Autodesk Fusion 360 part; units mm, degrees
(part 5 of 5)
  spline S268 degree 5 poles (-42.5645, -20.3407) (-42.5479, -20.3413) (-42.5148, -20.3422) (-42.4652, -20.3436) (-42.3991, -20.3453) (-42.3165, -20.347) (-42.234, -20.3485) (-42.1516, -20.3496) (-42.0693, -20.3504) (-41.987, -20.3508) (-41.9048, -20.3509) (-41.8227, -20.3507) (-41.7407, -20.3502) (-41.6588, -20.3493) (-41.5769, -20.3481) (-41.4952, -20.3465) (-41.4135, -20.3446) (-41.332, -20.3423) (-41.2505, -20.3398) (-41.1691, -20.3368) (-41.0878, -20.3335) (-41.0211, -20.3305) (-40.9707, -20.3281) (-40.9365, -20.3264) (-40.9186, -20.3254) (-40.9168, -20.3254) knots -1 -1 -1 -1 -1 -1 -0.985714 -0.971429 -0.957143 -0.942857 -0.928571 -0.914286 -0.9 -0.885714 -0.871429 -0.857143 -0.842857 -0.828571 -0.814286 -0.8 -0.785714 -0.771429 -0.757143 -0.742857 -0.728571 -0.714286 -0.712736 -0.712736 -0.712736 -0.712736 -0.712736 -0.712736
  arc A171 (-31.978, -19.3309) -> (-30.8526, -21.1319) centre (0.7975, -0.1016) ccw
  spline S269 degree 5 poles (-45.622, -12.0047) (-45.6059, -12.0083) (-45.5735, -12.0154) (-45.525, -12.0261) (-45.4604, -12.0401) (-45.3796, -12.0573) (-45.2989, -12.0742) (-45.2181, -12.0907) (-45.1374, -12.1069) (-45.0566, -12.1228) (-44.9759, -12.1383) (-44.8953, -12.1534) (-44.8146, -12.1683) (-44.734, -12.1828) (-44.6533, -12.1969) (-44.5727, -12.2107) (-44.4922, -12.2241) (-44.4116, -12.2372) (-44.3311, -12.2499) (-44.2506, -12.2623) (-44.1702, -12.2743) (-44.1041, -12.2838) (-44.0541, -12.2909) (-44.0202, -12.2956) (-44.0024, -12.2981) (-44.0007, -12.2983) knots -1 -1 -1 -1 -1 -1 -0.985714 -0.971429 -0.957143 -0.942857 -0.928571 -0.914286 -0.9 -0.885714 -0.871429 -0.857143 -0.842857 -0.828571 -0.814286 -0.8 -0.785714 -0.771429 -0.757143 -0.742857 -0.728571 -0.714286 -0.712736 -0.712736 -0.712736 -0.712736 -0.712736 -0.712736
  spline S270 degree 3 poles (-42.826, -15.9134) (-42.7781, -15.8674) (-42.7397, -15.8125) (-42.6859, -15.6911) (-42.6712, -15.6257) (-42.6676, -15.4929) (-42.6788, -15.4268) (-42.7258, -15.3026) (-42.7613, -15.2457) (-42.852, -15.1487) (-42.9064, -15.1095) (-43.0219, -15.0565) (-43.0811, -15.0413) (-43.1416, -15.0368) knots 0 0 0 0 0.019923 0.019923 0.039846 0.039846 0.059769 0.059769 0.079691 0.079691 0.099614 0.099614 0.117812 0.117812 0.117812 0.117812
  arc A172 (-44.9524, -14.3096) -> (-44.7782, -14.8456) centre (0, 0) ccw
  circle A173 centre (-9.5671, -23.097) radius 1.5
  arc A174 (-45.7622, -11.4588) -> (-45.622, -12.0047) centre (0, 0) ccw
  spline S271 degree 5 poles (-43.7577, -17.628) (-43.7412, -17.6295) (-43.7082, -17.6326) (-43.6588, -17.6371) (-43.5929, -17.6429) (-43.5106, -17.6498) (-43.4284, -17.6564) (-43.3462, -17.6627) (-43.264, -17.6686) (-43.182, -17.6743) (-43.1, -17.6795) (-43.018, -17.6845) (-42.9361, -17.6891) (-42.8543, -17.6933) (-42.7726, -17.6973) (-42.6909, -17.7008) (-42.6093, -17.7041) (-42.5277, -17.707) (-42.4462, -17.7095) (-42.3648, -17.7117) (-42.2835, -17.7135) (-42.2168, -17.7147) (-42.1663, -17.7154) (-42.1321, -17.7158) (-42.1141, -17.716) (-42.1123, -17.7161) knots -1 -1 -1 -1 -1 -1 -0.985714 -0.971429 -0.957143 -0.942857 -0.928571 -0.914286 -0.9 -0.885714 -0.871429 -0.857143 -0.842857 -0.828571 -0.814286 -0.8 -0.785714 -0.771429 -0.757143 -0.742857 -0.728571 -0.714286 -0.712736 -0.712736 -0.712736 -0.712736 -0.712736 -0.712736
  spline S272 degree 5 poles (-45.6475, -1.9006) (-45.6491, -1.9013) (-45.6653, -1.9092) (-45.6961, -1.9241) (-45.7414, -1.9463) (-45.8013, -1.9758) (-45.8741, -2.0121) (-45.9468, -2.0487) (-46.0195, -2.0857) (-46.092, -2.123) (-46.1645, -2.1607) (-46.2369, -2.1987) (-46.3092, -2.2371) (-46.3814, -2.2758) (-46.4536, -2.3148) (-46.5256, -2.3542) (-46.5976, -2.3938) (-46.6694, -2.4339) (-46.7412, -2.4742) (-46.8129, -2.5149) (-46.8845, -2.5559) (-46.956, -2.5972) (-47.0132, -2.6305) (-47.056, -2.6556) (-47.0845, -2.6724) (-47.0988, -2.6809) knots 0.712736 0.712736 0.712736 0.712736 0.712736 0.712736 0.714286 0.728571 0.742857 0.757143 0.771429 0.785714 0.8 0.814286 0.828571 0.842857 0.857143 0.871429 0.885714 0.9 0.914286 0.928571 0.942857 0.957143 0.971429 0.985714 1 1 1 1 1 1
  line L83 (-26.7765, -11.9199) -> (-34.1296, -15.0714)
  arc A175 (36.5058, -13.0984) -> (37.1761, -11.0832) centre (0.7975, -0.1016) ccw
  arc A176 (27.48, -13.8145) -> (28.2723, -12.1489) centre (0.7975, -0.1016) ccw
  line L84 (29.5656, -8.6104) -> (37.1761, -11.0832)
  line L85 (28.2723, -12.1489) -> (35.5129, -15.556)
  line L86 (28.9883, -10.3622) -> (36.5058, -13.0984)
  arc A177 (30.6543, -3.0291) -> (30.7778, -1.1887) centre (0.7975, -0.1016) ccw
  line L87 (30.7778, -1.1887) -> (38.7642, -1.6912)
  spline S273 degree 5 poles (39.9814, -25.0393) (39.973, -25.025) (39.9561, -24.9965) (39.9307, -24.9539) (39.8967, -24.8972) (39.8539, -24.8265) (39.8109, -24.7561) (39.7677, -24.6859) (39.7242, -24.616) (39.6805, -24.5463) (39.6366, -24.4768) (39.5924, -24.4076) (39.548, -24.3387) (39.5033, -24.27) (39.4585, -24.2015) (39.4133, -24.1333) (39.368, -24.0654) (39.3224, -23.9978) (39.2765, -23.9304) (39.2305, -23.8632) (39.1841, -23.7964) (39.1459, -23.7416) (39.1168, -23.7004) (39.097, -23.6724) (39.0866, -23.6578) (39.0856, -23.6563) knots -1 -1 -1 -1 -1 -1 -0.985714 -0.971429 -0.957143 -0.942857 -0.928571 -0.914286 -0.9 -0.885714 -0.871429 -0.857143 -0.842857 -0.828571 -0.814286 -0.8 -0.785714 -0.771429 -0.757143 -0.742857 -0.728571 -0.714286 -0.712736 -0.712736 -0.712736 -0.712736 -0.712736 -0.712736
  spline S274 degree 5 poles (36.3835, -27.6324) (36.3852, -27.6328) (36.4027, -27.6371) (36.4359, -27.6452) (36.485, -27.657) (36.5499, -27.6725) (36.6292, -27.6909) (36.7085, -27.7091) (36.7881, -27.7269) (36.8678, -27.7444) (36.9476, -27.7615) (37.0277, -27.7784) (37.1078, -27.7949) (37.1881, -27.8111) (37.2686, -27.827) (37.3492, -27.8426) (37.4299, -27.8579) (37.5108, -27.8729) (37.5918, -27.8875) (37.673, -27.9019) (37.7543, -27.916) (37.8358, -27.9297) (37.901, -27.9405) (37.95, -27.9484) (37.9827, -27.9536) (37.9991, -27.9562) knots 0.712736 0.712736 0.712736 0.712736 0.712736 0.712736 0.714286 0.728571 0.742857 0.757143 0.771429 0.785714 0.8 0.814286 0.828571 0.842857 0.857143 0.871429 0.885714 0.9 0.914286 0.928571 0.942857 0.957143 0.971429 0.985714 1 1 1 1 1 1
  arc A178 (32.1518, -21.5703) -> (33.3022, -19.7852) centre (0.7975, -0.1016) ccw
  spline S275 degree 5 poles (38.3303, -27.5003) (38.3228, -27.4856) (38.3077, -27.4561) (38.285, -27.4119) (38.2546, -27.3532) (38.2164, -27.28) (38.1779, -27.207) (38.1392, -27.1342) (38.1002, -27.0617) (38.0609, -26.9894) (38.0214, -26.9173) (37.9817, -26.8455) (37.9417, -26.7739) (37.9015, -26.7025) (37.861, -26.6314) (37.8202, -26.5605) (37.7792, -26.4899) (37.738, -26.4195) (37.6964, -26.3493) (37.6547, -26.2794) (37.6126, -26.2098) (37.5779, -26.1528) (37.5514, -26.1098) (37.5335, -26.0807) (37.524, -26.0654) (37.5231, -26.0639) knots -1 -1 -1 -1 -1 -1 -0.985714 -0.971429 -0.957143 -0.942857 -0.928571 -0.914286 -0.9 -0.885714 -0.871429 -0.857143 -0.842857 -0.828571 -0.814286 -0.8 -0.785714 -0.771429 -0.757143 -0.742857 -0.728571 -0.714286 -0.712736 -0.712736 -0.712736 -0.712736 -0.712736 -0.712736
  spline S276 degree 5 poles (27.9562, -37.9991) (27.9536, -37.9827) (27.9484, -37.95) (27.9405, -37.901) (27.9297, -37.8358) (27.916, -37.7543) (27.9019, -37.673) (27.8875, -37.5918) (27.8729, -37.5108) (27.8579, -37.4299) (27.8426, -37.3492) (27.827, -37.2686) (27.8111, -37.1881) (27.7949, -37.1078) (27.7784, -37.0277) (27.7615, -36.9476) (27.7444, -36.8678) (27.7269, -36.7881) (27.7091, -36.7085) (27.6909, -36.6292) (27.6725, -36.5499) (27.657, -36.485) (27.6452, -36.4359) (27.6371, -36.4027) (27.6328, -36.3852) (27.6324, -36.3835) knots -1 -1 -1 -1 -1 -1 -0.985714 -0.971429 -0.957143 -0.942857 -0.928571 -0.914286 -0.9 -0.885714 -0.871429 -0.857143 -0.842857 -0.828571 -0.814286 -0.8 -0.785714 -0.771429 -0.757143 -0.742857 -0.728571 -0.714286 -0.712736 -0.712736 -0.712736 -0.712736 -0.712736 -0.712736
  spline S277 degree 3 poles (26.0639, -37.5231) (26.0074, -37.4881) (25.9447, -37.4645) (25.8136, -37.4427) (25.7466, -37.4446) (25.6171, -37.4742) (25.5559, -37.5014) (25.4473, -37.5779) (25.401, -37.6264) (25.3296, -37.7384) (25.3052, -37.8008) (25.2826, -37.9259) (25.2826, -37.987) (25.2933, -38.0467) knots 0 0 0 0 0.019923 0.019923 0.039846 0.039846 0.059769 0.059769 0.079691 0.079691 0.099614 0.099614 0.117812 0.117812 0.117812 0.117812
  arc A179 (42.5645, -20.3407) -> (42.8044, -19.8308) centre (0, 0) ccw
  arc A180 (29.2138, -25.3308) -> (30.5789, -23.7039) centre (0.7975, -0.1016) ccw
  arc A181 (29.8528, -36.5279) -> (30.2871, -36.1687) centre (0, 0) ccw
  arc A182 (41.2033, -22.9733) -> (41.4748, -22.4794) centre (0, 0) ccw
  arc A183 (37.9991, -27.9562) -> (38.3303, -27.5003) centre (0, 0) ccw
  spline S278 degree 3 poles (40.9168, -20.3254) (40.8505, -20.3219) (40.7841, -20.3314) (40.6588, -20.3754) (40.601, -20.4094) (40.5018, -20.4977) (40.4613, -20.5511) (40.403, -20.6705) (40.3857, -20.7352) (40.3771, -20.8678) (40.3858, -20.9343) (40.4263, -21.0547) (40.4557, -21.1083) (40.4939, -21.1555) knots 0 0 0 0 0.019923 0.019923 0.039846 0.039846 0.059769 0.059769 0.079691 0.079691 0.099614 0.099614 0.117812 0.117812 0.117812 0.117812
  spline S279 degree 3 poles (38.0467, -25.2933) (37.9814, -25.2816) (37.9143, -25.2827) (37.7845, -25.3107) (37.7229, -25.3372) (37.6134, -25.4123) (37.5665, -25.4602) (37.4937, -25.5713) (37.4685, -25.6334) (37.4433, -25.7638) (37.4436, -25.8309) (37.4686, -25.9554) (37.4911, -26.0123) (37.5231, -26.0639) knots 0 0 0 0 0.019923 0.019923 0.039846 0.039846 0.059769 0.059769 0.079691 0.079691 0.099614 0.099614 0.117812 0.117812 0.117812 0.117812
  arc A184 (37.8532, -8.5204) -> (38.2656, -6.4371) centre (0.7975, -0.1016) ccw
  arc A185 (25.8277, -28.6934) -> (27.3859, -27.2504) centre (0.7975, -0.1016) ccw
  spline S280 degree 5 poles (39.5598, -22.8544) (39.5616, -22.8546) (39.5795, -22.8567) (39.6135, -22.8606) (39.6636, -22.8662) (39.73, -22.8733) (39.8109, -22.8817) (39.892, -22.8898) (39.9731, -22.8975) (40.0544, -22.9048) (40.1357, -22.9118) (40.2172, -22.9185) (40.2988, -22.9249) (40.3805, -22.9309) (40.4624, -22.9366) (40.5443, -22.942) (40.6263, -22.947) (40.7084, -22.9517) (40.7907, -22.9561) (40.873, -22.9602) (40.9554, -22.964) (41.0379, -22.9674) (41.104, -22.9699) (41.1536, -22.9716) (41.1867, -22.9727) (41.2033, -22.9733) knots 0.712736 0.712736 0.712736 0.712736 0.712736 0.712736 0.714286 0.728571 0.742857 0.757143 0.771429 0.785714 0.8 0.814286 0.828571 0.842857 0.857143 0.871429 0.885714 0.9 0.914286 0.928571 0.942857 0.957143 0.971429 0.985714 1 1 1 1 1 1
  line L88 (27.48, -13.8145) -> (34.5953, -17.4713)
  spline S281 degree 3 poles (36.3835, -27.6324) (36.319, -27.6166) (36.252, -27.6135) (36.1207, -27.6332) (36.0575, -27.6558) (35.9435, -27.7239) (35.8937, -27.7688) (35.8141, -27.8751) (35.785, -27.9355) (35.7517, -28.0641) (35.7477, -28.131) (35.7649, -28.2569) (35.7838, -28.3151) (35.8125, -28.3685) knots 0 0 0 0 0.019923 0.019923 0.039846 0.039846 0.059769 0.059769 0.079691 0.079691 0.099614 0.099614 0.117812 0.117812 0.117812 0.117812
  spline S282 degree 5 poles (41.4748, -22.4794) (41.4655, -22.4657) (41.4468, -22.4383) (41.4188, -22.3974) (41.3812, -22.3429) (41.3341, -22.2751) (41.2868, -22.2075) (41.2392, -22.1402) (41.1915, -22.0731) (41.1435, -22.0063) (41.0953, -21.9397) (41.0468, -21.8734) (40.9982, -21.8074) (40.9493, -21.7417) (40.9002, -21.6762) (40.8509, -21.6109) (40.8014, -21.546) (40.7516, -21.4813) (40.7016, -21.4169) (40.6514, -21.3528) (40.601, -21.289) (40.5594, -21.2368) (40.5278, -21.1974) (40.5063, -21.1708) (40.495, -21.1568) (40.4939, -21.1555) knots -1 -1 -1 -1 -1 -1 -0.985714 -0.971429 -0.957143 -0.942857 -0.928571 -0.914286 -0.9 -0.885714 -0.871429 -0.857143 -0.842857 -0.828571 -0.814286 -0.8 -0.785714 -0.771429 -0.757143 -0.742857 -0.728571 -0.714286 -0.712736 -0.712736 -0.712736 -0.712736 -0.712736 -0.712736
  spline S283 degree 5 poles (38.0467, -25.2933) (38.0485, -25.2936) (38.0662, -25.2968) (38.0999, -25.3028) (38.1496, -25.3115) (38.2154, -25.3229) (38.2956, -25.3363) (38.376, -25.3494) (38.4565, -25.3622) (38.5371, -25.3747) (38.6179, -25.3868) (38.6988, -25.3986) (38.7798, -25.41) (38.861, -25.4212) (38.9423, -25.432) (39.0237, -25.4425) (39.1053, -25.4527) (39.1869, -25.4626) (39.2687, -25.4721) (39.3506, -25.4813) (39.4327, -25.4903) (39.5148, -25.4989) (39.5806, -25.5055) (39.63, -25.5104) (39.663, -25.5135) (39.6795, -25.5151) knots 0.712736 0.712736 0.712736 0.712736 0.712736 0.712736 0.714286 0.728571 0.742857 0.757143 0.771429 0.785714 0.8 0.814286 0.828571 0.842857 0.857143 0.871429 0.885714 0.9 0.914286 0.928571 0.942857 0.957143 0.971429 0.985714 1 1 1 1 1 1
  spline S284 degree 5 poles (40.9168, -20.3254) (40.9186, -20.3254) (40.9365, -20.3264) (40.9707, -20.3281) (41.0211, -20.3305) (41.0878, -20.3335) (41.1691, -20.3368) (41.2505, -20.3398) (41.332, -20.3423) (41.4135, -20.3446) (41.4952, -20.3465) (41.5769, -20.3481) (41.6588, -20.3493) (41.7407, -20.3502) (41.8227, -20.3507) (41.9048, -20.3509) (41.987, -20.3508) (42.0693, -20.3504) (42.1516, -20.3496) (42.234, -20.3485) (42.3165, -20.347) (42.3991, -20.3453) (42.4652, -20.3436) (42.5148, -20.3422) (42.5479, -20.3413) (42.5645, -20.3407) knots 0.712736 0.712736 0.712736 0.712736 0.712736 0.712736 0.714286 0.728571 0.742857 0.757143 0.771429 0.785714 0.8 0.814286 0.828571 0.842857 0.857143 0.871429 0.885714 0.9 0.914286 0.928571 0.942857 0.957143 0.971429 0.985714 1 1 1 1 1 1
  spline S285 degree 5 poles (36.5279, -29.8528) (36.5213, -29.8376) (36.5081, -29.8073) (36.4883, -29.7618) (36.4616, -29.7012) (36.4281, -29.6258) (36.3942, -29.5505) (36.3601, -29.4755) (36.3258, -29.4006) (36.2911, -29.326) (36.2563, -29.2516) (36.2211, -29.1774) (36.1857, -29.1034) (36.15, -29.0297) (36.1141, -28.9562) (36.0778, -28.8829) (36.0414, -28.8098) (36.0046, -28.7369) (35.9676, -28.6643) (35.9303, -28.5919) (35.8927, -28.5198) (35.8616, -28.4607) (35.8379, -28.4161) (35.8218, -28.3859) (35.8133, -28.3701) (35.8125, -28.3685) knots -1 -1 -1 -1 -1 -1 -0.985714 -0.971429 -0.957143 -0.942857 -0.928571 -0.914286 -0.9 -0.885714 -0.871429 -0.857143 -0.842857 -0.828571 -0.814286 -0.8 -0.785714 -0.771429 -0.757143 -0.742857 -0.728571 -0.714286 -0.712736 -0.712736 -0.712736 -0.712736 -0.712736 -0.712736
  arc A186 (25.5509, -17.0506) -> (26.5457, -15.4974) centre (0.7975, -0.1016) ccw
  arc A187 (39.6795, -25.5151) -> (39.9814, -25.0393) centre (0, 0) ccw
  spline S286 degree 3 poles (39.5598, -22.8544) (39.4939, -22.8468) (39.427, -22.8522) (39.2992, -22.8882) (39.2394, -22.9185) (39.1348, -23.0004) (39.091, -23.0511) (39.0253, -23.1666) (39.0041, -23.2302) (38.9871, -23.3619) (38.9916, -23.4288) (39.0245, -23.5515) (39.0505, -23.6069) (39.0856, -23.6563) knots 0 0 0 0 0.019923 0.019923 0.039846 0.039846 0.059769 0.059769 0.079691 0.079691 0.099614 0.099614 0.117812 0.117812 0.117812 0.117812
  arc A188 (30.052, -6.7481) -> (30.4052, -4.9377) centre (0.7975, -0.1016) ccw
  arc A189 (38.6162, -3.8098) -> (38.7642, -1.6912) centre (0.7975, -0.1016) ccw
  line L89 (30.6543, -3.0291) -> (38.6162, -3.8098)
  line L90 (30.052, -6.7481) -> (37.8532, -8.5204)
  line L91 (30.4052, -4.9377) -> (38.2656, -6.4371)
  arc A190 (28.9883, -10.3622) -> (29.5656, -8.6104) centre (0.7975, -0.1016) ccw
  arc A191 (34.5953, -17.4713) -> (35.5129, -15.556) centre (0.7975, -0.1016) ccw
  arc A192 (17.9309, -34.0199) -> (19.799, -33.0097) centre (0.7975, -0.1016) ccw
  arc A193 (10.8611, -28.3633) -> (12.5789, -27.6915) centre (0.7975, -0.1016) ccw
  line L92 (9.028, -28.9505) -> (11.0181, -36.7013)
  line L93 (7.2396, -29.4018) -> (8.9575, -37.2151)
  circle A194 centre (23.097, -9.5671) radius 1.5
  arc A195 (13.5447, -35.8998) -> (15.5247, -35.1317) centre (0.7975, -0.1016) ccw
  line L94 (5.3474, -29.7546) -> (6.3503, -37.6937)
  line L95 (3.5165, -29.9781) -> (4.2415, -37.9452)
  arc A196 (17.5733, -24.9727) -> (19.07, -23.8948) centre (0.7975, -0.1016) ccw
  arc A197 (7.2396, -29.4018) -> (9.028, -28.9505) centre (0.7975, -0.1016) ccw
  line L96 (10.8611, -28.3633) -> (13.5447, -35.8998)
  line L97 (17.5733, -24.9727) -> (22.0468, -31.605)
  line L98 (12.5789, -27.6915) -> (15.5247, -35.1317)
  arc A198 (14.3238, -26.8792) -> (15.9439, -25.9973) centre (0.7975, -0.1016) ccw
  arc A199 (20.5582, -22.674) -> (21.908, -21.417) centre (0.7975, -0.1016) ccw
  line L99 (14.3238, -26.8792) -> (17.9309, -34.0199)
  arc A200 (23.2315, -20.0194) -> (24.4131, -18.6031) centre (0.7975, -0.1016) ccw
  line L100 (15.9439, -25.9973) -> (19.799, -33.0097)
  line L101 (-0.2495, -30.0833) -> (-0.5287, -38.0785)
  line L102 (1.595, -30.091) -> (1.595, -38.0932)
  arc A201 (25.0393, -39.9814) -> (25.5151, -39.6795) centre (0, 0) ccw
  arc A202 (36.1687, -30.2871) -> (36.5279, -29.8528) centre (0, 0) ccw
  spline S287 degree 5 poles (32.4983, -34.1956) (32.4937, -34.1797) (32.4844, -34.1479) (32.4704, -34.1003) (32.4516, -34.0369) (32.4277, -33.9578) (32.4036, -33.8789) (32.3792, -33.8002) (32.3544, -33.7216) (32.3295, -33.6433) (32.3042, -33.5651) (32.2786, -33.4871) (32.2527, -33.4092) (32.2266, -33.3316) (32.2001, -33.2541) (32.1734, -33.1769) (32.1463, -33.0998) (32.119, -33.0229) (32.0914, -32.9462) (32.0634, -32.8697) (32.0352, -32.7934) (32.0117, -32.7309) (31.9938, -32.6837) (31.9816, -32.6518) (31.9752, -32.635) (31.9746, -32.6333) knots -1 -1 -1 -1 -1 -1 -0.985714 -0.971429 -0.957143 -0.942857 -0.928571 -0.914286 -0.9 -0.885714 -0.871429 -0.857143 -0.842857 -0.828571 -0.814286 -0.8 -0.785714 -0.771429 -0.757143 -0.742857 -0.728571 -0.714286 -0.712736 -0.712736 -0.712736 -0.712736 -0.712736 -0.712736
  spline S288 degree 5 poles (34.5766, -29.8624) (34.5783, -29.8629) (34.5955, -29.8683) (34.6281, -29.8785) (34.6764, -29.8934) (34.7402, -29.9128) (34.8182, -29.9362) (34.8962, -29.9593) (34.9745, -29.9821) (35.053, -30.0046) (35.1316, -30.0267) (35.2104, -30.0485) (35.2893, -30.0701) (35.3685, -30.0913) (35.4478, -30.1122) (35.5272, -30.1329) (35.6069, -30.1532) (35.6866, -30.1732) (35.7666, -30.1929) (35.8467, -30.2124) (35.927, -30.2315) (36.0074, -30.2503) (36.0718, -30.2652) (36.1202, -30.2762) (36.1525, -30.2834) (36.1687, -30.2871) knots 0.712736 0.712736 0.712736 0.712736 0.712736 0.712736 0.714286 0.728571 0.742857 0.757143 0.771429 0.785714 0.8 0.814286 0.828571 0.842857 0.857143 0.871429 0.885714 0.9 0.914286 0.928571 0.942857 0.957143 0.971429 0.985714 1 1 1 1 1 1
  spline S289 degree 3 poles (28.3685, -35.8125) (28.31, -35.7811) (28.2459, -35.7615) (28.1138, -35.7479) (28.047, -35.7541) (27.9196, -35.7917) (27.8602, -35.8228) (27.7566, -35.9059) (27.7135, -35.9572) (27.6492, -36.0735) (27.6288, -36.1373) (27.6141, -36.2635) (27.6179, -36.3246) (27.6324, -36.3835) knots 0 0 0 0 0.019923 0.019923 0.039846 0.039846 0.059769 0.059769 0.079691 0.079691 0.099614 0.099614 0.117812 0.117812 0.117812 0.117812
  spline S290 degree 5 poles (26.0639, -37.5231) (26.0654, -37.524) (26.0807, -37.5335) (26.1098, -37.5514) (26.1528, -37.5779) (26.2098, -37.6126) (26.2794, -37.6547) (26.3493, -37.6964) (26.4195, -37.738) (26.4899, -37.7792) (26.5605, -37.8202) (26.6314, -37.861) (26.7025, -37.9015) (26.7739, -37.9417) (26.8455, -37.9817) (26.9173, -38.0214) (26.9894, -38.0609) (27.0617, -38.1002) (27.1342, -38.1392) (27.207, -38.1779) (27.28, -38.2164) (27.3532, -38.2546) (27.4119, -38.285) (27.4561, -38.3077) (27.4856, -38.3228) (27.5003, -38.3303) knots 0.712736 0.712736 0.712736 0.712736 0.712736 0.712736 0.714286 0.728571 0.742857 0.757143 0.771429 0.785714 0.8 0.814286 0.828571 0.842857 0.857143 0.871429 0.885714 0.9 0.914286 0.928571 0.942857 0.957143 0.971429 0.985714 1 1 1 1 1 1
  spline S291 degree 5 poles (25.5151, -39.6795) (25.5135, -39.663) (25.5104, -39.63) (25.5055, -39.5806) (25.4989, -39.5148) (25.4903, -39.4327) (25.4813, -39.3506) (25.4721, -39.2687) (25.4626, -39.1869) (25.4527, -39.1053) (25.4425, -39.0237) (25.432, -38.9423) (25.4212, -38.861) (25.41, -38.7798) (25.3986, -38.6988) (25.3868, -38.6179) (25.3747, -38.5371) (25.3622, -38.4565) (25.3494, -38.376) (25.3363, -38.2956) (25.3229, -38.2154) (25.3115, -38.1496) (25.3028, -38.0999) (25.2968, -38.0662) (25.2936, -38.0485) (25.2933, -38.0467) knots -1 -1 -1 -1 -1 -1 -0.985714 -0.971429 -0.957143 -0.942857 -0.928571 -0.914286 -0.9 -0.885714 -0.871429 -0.857143 -0.842857 -0.828571 -0.814286 -0.8 -0.785714 -0.771429 -0.757143 -0.742857 -0.728571 -0.714286 -0.712736 -0.712736 -0.712736 -0.712736 -0.712736 -0.712736
  arc A203 (32.0875, -34.5814) -> (32.4983, -34.1956) centre (0, 0) ccw
  spline S292 degree 3 poles (32.6333, -31.9746) (32.5713, -31.9508) (32.5053, -31.9393) (32.3725, -31.9424) (32.307, -31.9569) (32.1854, -32.0102) (32.1303, -32.0485) (32.038, -32.144) (32.0016, -32.2003) (31.9524, -32.3237) (31.9401, -32.3896) (31.9414, -32.5166) (31.9528, -32.5767) (31.9746, -32.6333) knots 0 0 0 0 0.019923 0.019923 0.039846 0.039846 0.059769 0.059769 0.079691 0.079691 0.099614 0.099614 0.117812 0.117812 0.117812 0.117812
  spline S293 degree 5 poles (28.3685, -35.8125) (28.3701, -35.8133) (28.3859, -35.8218) (28.4161, -35.8379) (28.4607, -35.8616) (28.5198, -35.8927) (28.5919, -35.9303) (28.6643, -35.9676) (28.7369, -36.0046) (28.8098, -36.0414) (28.8829, -36.0778) (28.9562, -36.1141) (29.0297, -36.15) (29.1034, -36.1857) (29.1774, -36.2211) (29.2516, -36.2563) (29.326, -36.2911) (29.4006, -36.3258) (29.4755, -36.3601) (29.5505, -36.3942) (29.6258, -36.4281) (29.7012, -36.4616) (29.7618, -36.4883) (29.8073, -36.5081) (29.8376, -36.5213) (29.8528, -36.5279) knots 0.712736 0.712736 0.712736 0.712736 0.712736 0.712736 0.714286 0.728571 0.742857 0.757143 0.771429 0.785714 0.8 0.814286 0.828571 0.842857 0.857143 0.871429 0.885714 0.9 0.914286 0.928571 0.942857 0.957143 0.971429 0.985714 1 1 1 1 1 1
  spline S294 degree 5 poles (30.5612, -33.9605) (30.5628, -33.9613) (30.5792, -33.9687) (30.6103, -33.9829) (30.6563, -34.0037) (30.7172, -34.0311) (30.7916, -34.0641) (30.8662, -34.0967) (30.941, -34.1291) (31.016, -34.1613) (31.0912, -34.1931) (31.1666, -34.2246) (31.2423, -34.2559) (31.3181, -34.2869) (31.3942, -34.3176) (31.4704, -34.348) (31.5469, -34.3781) (31.6235, -34.408) (31.7004, -34.4376) (31.7774, -34.4669) (31.8546, -34.496) (31.9321, -34.5247) (31.9942, -34.5475) (32.0408, -34.5645) (32.0719, -34.5758) (32.0875, -34.5814) knots 0.712736 0.712736 0.712736 0.712736 0.712736 0.712736 0.714286 0.728571 0.742857 0.757143 0.771429 0.785714 0.8 0.814286 0.828571 0.842857 0.857143 0.871429 0.885714 0.9 0.914286 0.928571 0.942857 0.957143 0.971429 0.985714 1 1 1 1 1 1
  arc A204 (34.1956, -32.4983) -> (34.5814, -32.0875) centre (0, 0) ccw
  arc A205 (27.5003, -38.3303) -> (27.9562, -37.9991) centre (0, 0) ccw
  spline S295 degree 5 poles (34.5814, -32.0875) (34.5758, -32.0719) (34.5645, -32.0408) (34.5475, -31.9942) (34.5247, -31.9321) (34.496, -31.8546) (34.4669, -31.7774) (34.4376, -31.7004) (34.408, -31.6235) (34.3781, -31.5469) (34.348, -31.4704) (34.3176, -31.3942) (34.2869, -31.3181) (34.2559, -31.2423) (34.2246, -31.1666) (34.1931, -31.0912) (34.1613, -31.016) (34.1291, -30.941) (34.0967, -30.8662) (34.0641, -30.7916) (34.0311, -30.7172) (34.0037, -30.6563) (33.9829, -30.6103) (33.9687, -30.5792) (33.9613, -30.5628) (33.9605, -30.5612) knots -1 -1 -1 -1 -1 -1 -0.985714 -0.971429 -0.957143 -0.942857 -0.928571 -0.914286 -0.9 -0.885714 -0.871429 -0.857143 -0.842857 -0.828571 -0.814286 -0.8 -0.785714 -0.771429 -0.757143 -0.742857 -0.728571 -0.714286 -0.712736 -0.712736 -0.712736 -0.712736 -0.712736 -0.712736
  spline S296 degree 3 poles (30.5612, -33.9605) (30.5008, -33.9329) (30.4356, -33.9173) (30.3029, -33.9121) (30.2367, -33.9225) (30.1119, -33.968) (30.0546, -34.0027) (29.9564, -34.0922) (29.9166, -34.1461) (29.8597, -34.2662) (29.8433, -34.3312) (29.8366, -34.4581) (29.8443, -34.5187) (29.8624, -34.5766) knots 0 0 0 0 0.019923 0.019923 0.039846 0.039846 0.059769 0.059769 0.079691 0.079691 0.099614 0.099614 0.117812 0.117812 0.117812 0.117812
  spline S297 degree 5 poles (30.2871, -36.1687) (30.2834, -36.1525) (30.2762, -36.1202) (30.2652, -36.0718) (30.2503, -36.0074) (30.2315, -35.927) (30.2124, -35.8467) (30.1929, -35.7666) (30.1732, -35.6866) (30.1532, -35.6069) (30.1329, -35.5272) (30.1122, -35.4478) (30.0913, -35.3685) (30.0701, -35.2893) (30.0485, -35.2104) (30.0267, -35.1316) (30.0046, -35.053) (29.9821, -34.9745) (29.9593, -34.8962) (29.9362, -34.8182) (29.9128, -34.7402) (29.8934, -34.6764) (29.8785, -34.6281) (29.8683, -34.5955) (29.8629, -34.5783) (29.8624, -34.5766) knots -1 -1 -1 -1 -1 -1 -0.985714 -0.971429 -0.957143 -0.942857 -0.928571 -0.914286 -0.9 -0.885714 -0.871429 -0.857143 -0.842857 -0.828571 -0.814286 -0.8 -0.785714 -0.771429 -0.757143 -0.742857 -0.728571 -0.714286 -0.712736 -0.712736 -0.712736 -0.712736 -0.712736 -0.712736
  spline S298 degree 5 poles (32.6333, -31.9746) (32.635, -31.9752) (32.6518, -31.9816) (32.6837, -31.9938) (32.7309, -32.0117) (32.7934, -32.0352) (32.8697, -32.0634) (32.9462, -32.0914) (33.0229, -32.119) (33.0998, -32.1463) (33.1769, -32.1734) (33.2541, -32.2001) (33.3316, -32.2266) (33.4092, -32.2527) (33.4871, -32.2786) (33.5651, -32.3042) (33.6433, -32.3295) (33.7216, -32.3544) (33.8002, -32.3792) (33.8789, -32.4036) (33.9578, -32.4277) (34.0369, -32.4516) (34.1003, -32.4704) (34.1479, -32.4844) (34.1797, -32.4937) (34.1956, -32.4983) knots 0.712736 0.712736 0.712736 0.712736 0.712736 0.712736 0.714286 0.728571 0.742857 0.757143 0.771429 0.785714 0.8 0.814286 0.828571 0.842857 0.857143 0.871429 0.885714 0.9 0.914286 0.928571 0.942857 0.957143 0.971429 0.985714 1 1 1 1 1 1
  spline S299 degree 3 poles (34.5766, -29.8624) (34.5132, -29.8426) (34.4466, -29.8353) (34.3143, -29.8467) (34.2499, -29.8653) (34.1318, -29.9261) (34.0792, -29.9678) (33.9931, -30.0689) (33.9603, -30.1273) (33.919, -30.2536) (33.9108, -30.3201) (33.9201, -30.4468) (33.9353, -30.5061) (33.9605, -30.5612) knots 0 0 0 0 0.019923 0.019923 0.039846 0.039846 0.059769 0.059769 0.079691 0.079691 0.099614 0.099614 0.117812 0.117812 0.117812 0.117812
  line L103 (-17.0171, -1.5465) -> (-10.5309, -1.4899)
  line L104 (17.068, -1.5604) -> (10.5293, -1.5017)
  circle A206 centre (19, 0.0262) radius 2.5
  circle A207 centre (-23.097, 9.5671) radius 1.5
  circle A208 centre (0, 0) radius 32
  arc A209 (-10.9644, 13.1731) -> (-13.1272, 10.9389) centre (-13.4524, 13.4176) ccw
  line L105 (-13.1731, -10.9644) -> (-7.3425, -5.2295)
  line L106 (17.017, 1.5486) -> (10.5308, 1.4912)
  circle A210 centre (0, 0) radius 1.5
  line L107 (0, 0) -> (0.0807, -19)
  arc A211 (-17.0678, 1.5625) -> (-17.0171, -1.5465) centre (-19, -0.0239) ccw
  circle A212 centre (23.097, -9.5671) radius 1.5
  line L108 (10.9661, -13.1716) -> (5.2305, -7.3416)
  line L109 (1.5604, 17.068) -> (1.5017, 10.5293)
  line L110 (1.5836, -17.0022) -> (1.4815, -8.8772)
  line L111 (-17.0678, 1.5625) -> (-10.5294, 1.503)
  line L112 (-10.9389, -13.1272) -> (-5.239, -7.3351)
  line L113 (10.9372, 13.1287) -> (5.2381, 7.336)
  arc A213 (-13.1731, -10.9644) -> (-10.9389, -13.1272) centre (-13.4176, -13.4524) ccw
  line L114 (-13.1272, 10.9389) -> (-7.3351, 5.239)
  line L115 (-1.5486, 17.017) -> (-1.4912, 10.5308)
  line L116 (-1.6201, -17.1677) -> (-1.6201, -8.853)
  circle A214 centre (-9.5671, -23.097) radius 1.5
  circle A215 centre (13.4159, 13.4541) radius 2.5
  line L117 (-10.9644, 13.1731) -> (-5.2295, 7.3425)
  line L118 (13.1716, 10.9661) -> (7.3416, 5.2305)
  circle A216 centre (9.5671, 23.097) radius 1.5
  line L119 (13.1287, -10.9372) -> (7.336, -5.2381)
  circle A217 centre (13.4541, -13.4159) radius 2.5
  circle A218 centre (0, 0) radius 9
  circle A219 centre (0.0807, -19) radius 2.5
  circle A220 centre (0, 0) radius 11
  circle A221 centre (0, 0) radius 25
  circle A222 centre (-0.0262, 19) radius 2.5
  dimension "d2" = 360
  dimension "d86" = 76
  dimension "d87" = 88
  dimension "d6" = 360
  dimension "d8" = 360
  dimension "d10" = 5
  dimension "d12" = 18
  dimension "d17" = 64
  dimension "d18" = 50
  dimension "d19" = 3
  dimension "d22" = 22
  dimension "d42" = 19
  dimension "d43" = 19
  dimension "d45" = 19
  dimension "d46" = 19
  dimension "d47" = 19
  dimension "d48" = 19
  dimension "d49" = 19
  dimension "d50" = 19
  constraint coincident A1.centre A2.centre
  constraint vertical L8
  constraint horizontal L61
  constraint coincident A0.centre A3.centre
  constraint coincident L7.end A1
  constraint collinear L7 L15
  constraint coincident L8.end A1
  constraint collinear L8 L12
  constraint vertical L116
  constraint coincident L116.end A218
  constraint coincident L110.end A218
  constraint coincident A173.centre A221
  constraint coincident L116.start A219
  constraint coincident L110.start A219
  constraint coincident L115.start A222
  constraint coincident L109.start A222
  constraint coincident L118.start A215
  constraint coincident L113.start A215
  constraint coincident L104.start A206
  constraint coincident L106.start A206
  constraint coincident L108.start A217
  constraint coincident L119.start A217
  constraint coincident L107.end A219.centre
  measures "d86" diameter of A39
  measures "d87" angle of L7 L61
  measures "d10" diameter of A219
  measures "d12" diameter of A218
  measures "d17" diameter of A208
  measures "d18" diameter of A221
  measures "d19" diameter of A214
  measures "d22" diameter of A220
  measures "d42" vertical distance of A1.centre L107.end
  measures "d43" distance of A1.centre A213.centre
  measures "d45" horizontal distance of A1.centre A211.centre
  measures "d46" distance of A1.centre A209.centre
  measures "d47" vertical distance of A1.centre A222.centre
  measures "d48" distance of A1.centre A215.centre
  measures "d49" horizontal distance of A1.centre A206.centre
  measures "d50" distance of A217.centre A1.centre
extrude "Extrude1" add sketch "Sketch1" along normal blind 8 contours S0 S1 S2 S3 S4 S5 S6 A4 S7 A5 S8 S9 S10 S11 S12 S13 S14 A6 S15 S16 A8 S17 A9 S18 S19 S20 A10 S21 A11 S22 S23 A13 S24 S25 S26 A14 S27 S28 S29 S30 A17 S31 S32 A18 S33 A19 S34 S35 S36 A20 S37 S38 S39 S40 S41 S42 S43 A21 S44 S45 S46 S47 A22 S48 S49 S50 S51 A30 S52 A53 S53 S54 A58 A59 S55 S56 S57 A60 S58 S59 S60 S61 A62 S62 S63 S64 A66 S65 S66 S67 S68 S69 A69 S70 S71 S72 S73 S74 S75 S76 S77 S78 S79 S80 A73 S81 S82 S83 A75 S84 S85 S86 S87 S88 A77 A78 S89 S90 S91 A80 S92 S93 S94 S95 S96 S97 A81 S98 S99 S100 S101 S102 A82 S103 S104 S105 S106 S107 S108 S109 A84 S110 S111 S112 S113 A86 S114 S115 S116 A88 S117 S118 S119 A89 A90 A91 S120 S121 S122 S123 S124 S125 S126 S127 A93 S128 A94 A95 S129 S130 S131 S132 A96 A98 S133 A100 S134 A101 S135 S136 S137 S138 S139 A102 S140 S141 S142 S143 S144 S145 S146 S147 A103 A104 S148 S149 A105 S150 S151 A106 S152 S153 S154 A108 S155 S156 A110 S157 A112 S158 S159 A113 S160 S161 A116 S162 S163 S164 S165 A118 S166 S167 S168 S169 A120 S170 S171 S172 S173 S174 S175 A123 S176 S177 A124 S178 S179 A125 S180 S181 S182 S183 S184 S185 S186 S187 S188 A126 S189 S190 S191 S192 S193 S194 A127 S195 S196 S197 A128 A129 S198 S199 S200 A131 S201 S202 S203 S204 S205 S206 A132 A133 A134 S207 S208 S209 S210 A135 S211 A136 S212 A137 S213 A138 S214 S215 S216 S217 A140 S218 S219 S220 S221 S222 S223 A141 A142 A143 A144 A145 S224 S225 S226 S227 S228 S229 S230 A147 S231 S232 S233 S234 S235 S236 S237 S238 A152 S239 S240 S241 S242 A153 S243 S244 S245 A154 S246 S247 S248 S249 S250 A156 A157 S251 S252 A158 S253 S254 A162 S255 S256 S257 A163 S258 A164 S259 S260 A168 S261 S262 S263 S264 A169 S265 S266 S267 S268 S269 S270 A172 A174 S271 S272 S273 S274 S275 S276 S277 A179 A181 A182 A183 S278 S279 S280 S281 S282 S283 S284 S285 A187 S286 A201 A202 S287 S288 S289 S290 S291 A203 S292 S293 S294 A204 A205 S295 S296 S297 S298 S299 | A3 A15 L0 L1 L2 L3 L4 L5 L6 A24 A25 A26 A27 A28 A29 A31 L9 L10 L11 L12 L13 L14 L15 L16 A34 A36 L17 L18 L19 A38 A40 A41 L20 A43 L21 L22 L23 A48 A49 L24 L25 L26 L27 A50 L28 L29 L30 L31 L32 L33 L34 A54 A55 L35 L36 A56 L37 L38 A61 L39 L40 L41 L42 L43 L44 A63 L45 L46 A64 L47 L48 A68 L49 L50 L51 L52 A72 L53 L54 A83 A85 L55 L56 L57 L58 A107 L59 L60 L62 L63 A115 L64 L65 L66 L67 A119 L68 L69 L70 L71 L72 L73 A146 L74 A148 L75 A149 A150 A151 A160 L76 L77 L78 A166 L79 A170 L80 L81 L82 L83 A176 L84 L85 L86 A177 L87 L88 A186 A188 L89 L90 L91 A190 A193 L92 L93 L94 L95 A196 A197 L96 L97 L98 A198 A199 L99 A200 L100 L101 L102 A208 | A23 A45 A173 A194 A207 A212 A214 A216 A221
equation "d42 = r1"
equation "d43 = r1"
equation "d45 = r1"
equation "d46 = r1"
equation "d47 = r1"
equation "d48 = r1"
equation "d49 = r1"
equation "d50 = r1"
